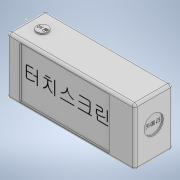
# Autodesk Inventor part: 구상도
Saved by Autodesk Inventor 2022.1 (Build 261234000, 234)
## iProperties
Created: 2021-09-09
Part Number: 구상도
Material: 일반
Document SubType Name: Modeling
Designer: jwchu
Density: 1 g/cm^3
Appearance: 기본값
Author: jwchu
Autodesk Inventor part; units mm, degrees
ref_plane "YZ Plane" through (0, 0, 0) normal (1, 0, 0) x (0, 1, 0)
ref_plane "XZ Plane" through (0, 0, 0) normal (0, 1, 0) x (-1, 0, 0)
ref_plane "XY Plane" through (0, 0, 0) normal (0, 0, 1) x (1, 0, 0)
sketch "스케치1" plane through (0, 0, 0) normal (0, 0, 1) x (1, 0, 0)
  line L0 (0, 0) -> (100, 0)
  line L1 (100, 0) -> (100, 45)
  line L2 (100, 45) -> (0, 45)
  line L3 (0, 45) -> (0, 0)
  dimension "d0" = 100
  dimension "d1" = 45
  constraints: 8 end point, 2 parallel, 1 horizontal, 1 perpendicular
  measures "d0" distance of L2.end L1.end
  measures "d1" distance of L1.end L0.end
extrude "돌출1" add sketch "스케치1" along normal mid plane 30
sketch "스케치2" plane through (100, 0, 15) normal (1, 0, 0) x (0, 0, -1)
  circle A0 centre (15, 24.5901) radius 7.5
  point P0 (15, 0)
  dimension "d4" = 15
  constraints: 1 centre point
  measures "d4" diameter of A0
extrude "돌출2" cut sketch "스케치2" against normal blind 1
sketch "스케치3" plane through (0, 0, 15) normal (0, 0, 1) x (1, 0, 0)
  line L0 (10, 42.5) -> (80, 42.5)
  line L1 (80, 42.5) -> (80, 2.5)
  line L2 (80, 2.5) -> (10, 2.5)
  line L3 (10, 2.5) -> (10, 42.5)
  line L4 (100, 45) -> (0, 45) projected
  line L5 (0, 45) -> (0, 0) projected
  dimension "d7" = 70
  dimension "d8" = 40
  dimension "d9" = 2.5
  dimension "d10" = 10
  constraints: 8 end point, 2 parallel, 1 horizontal, 1 perpendicular
  measures "d7" distance of L1.end L2.end
  measures "d8" distance of L0.end L1.end
  measures "d9" distance between parallel lines of L0 L4
  measures "d10" distance between parallel lines of L3 L5
extrude "돌출3" cut sketch "스케치3" against normal blind 1
sketch "스케치4" plane through (0, 0, 14) normal (0, 0, 1) x (1, 0, 0)
  line L0 (11.7603, 30.0874) -> (53.0164, 30.0874) construction
  line L1 (53.0164, 30.0874) -> (53.0164, 23.3337) construction
  line L2 (53.0164, 23.3337) -> (11.7603, 23.3337) construction
  line L3 (11.7603, 23.3337) -> (11.7603, 30.0874) construction
  point P0 (0, 0)
  constraints: 2 other
sketch "스케치5" plane through (99, 24.5901, 0) normal (1, 0, 0) x (0, 0, -1)
  line L0 (-5.91, 1.6766) -> (6.6648, 1.6766) construction
  line L1 (6.6648, 1.6766) -> (6.6648, -1.7518) construction
  line L2 (6.6648, -1.7518) -> (-5.91, -1.7518) construction
  line L3 (-5.91, -1.7518) -> (-5.91, 1.6766) construction
  point P0 (0, -24.5901)
  constraints: 2 other
sketch "스케치6" plane through (0, 45, 15) normal (0, 1, 0) x (1, 0, 0)
  circle A0 centre (12.5978, 15) radius 4.3939
  point P0 (0, 15)
  constraints: 1 centre point
extrude "돌출4" add sketch "스케치6" along normal blind 1
sketch "스케치7" plane through (12.5978, 46, 0) normal (0, 1, 0) x (1, 0, 0)
  line L0 (-4.0633, 1.8765) -> (4.3199, 1.8765) construction
  line L1 (4.3199, 1.8765) -> (4.3199, -1.5495) construction
  line L2 (4.3199, -1.5495) -> (-4.0633, -1.5495) construction
  line L3 (-4.0633, -1.5495) -> (-4.0633, 1.8765) construction
  point P0 (-12.5978, 0)
  constraints: 2 other
fillet "모깎기1" radius 2 11 edges at (50, 45, 15) (100, 45, 0) (100, 22.5, 15) (100, 22.5, -15) (50, 45, -15) (50, 0, -15) (50, 0, 15) (100, 0, 0) (0, 0, 0) (0, 22.5, 15) (0, 22.5, -15)
fillet "모깎기2" radius 2 3 edges at (0, 45, 0) (0.5858, 44.4142, 14.4142) (0.5858, 44.4142, -14.4142)
